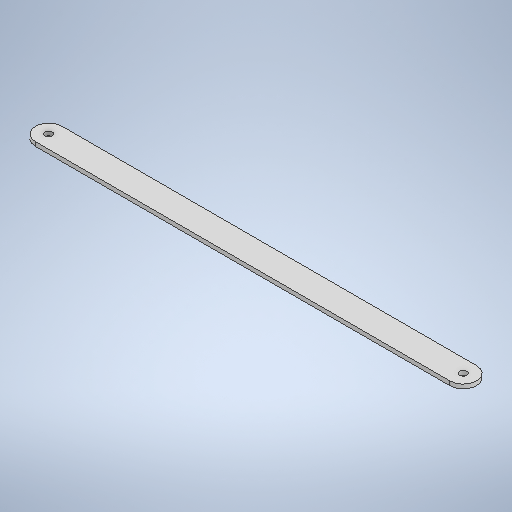
# Autodesk Inventor part: A1P2
Saved by Autodesk Inventor 2025.2 (Build 292293000, 293)
## iProperties
Created: 2025-05-22
Part Number: A1P2
Material: Generic
Document SubType Name: Sheet Metal
Designer: Admin
Density: 1 g/cm^3
Sheet Metal Rule: Default
Appearance: Default
Author: Admin
Autodesk Inventor part; units mm, degrees
ref_plane "YZ Plane" through (0, 0, 0) normal (1, 0, 0) x (0, 1, 0)
ref_plane "XZ Plane" through (0, 0, 0) normal (0, 1, 0) x (-1, 0, 0)
ref_plane "XY Plane" through (0, 0, 0) normal (0, 0, 1) x (1, 0, 0)
sketch "Sketch1" plane through (0, 0, 0) normal (0, 1, 0) x (-1, 0, 0)
  arc A0 (0, 5.4545) -> (0, -5.4545) centre (0, 0) ccw
  arc A1 (170, -5.4545) -> (170, 5.4545) centre (170, 0) ccw
  line L0 (0, 5.4545) -> (170, 5.4545)
  line L1 (170, -5.4545) -> (0, -5.4545)
  dimension "d0" = 10.909
  dimension "d1" = 10.909
  dimension "d2" = 170
  constraints: 4 end point, 4 point on circle, 4 tangent, 2 centre point, 1 coincident
  measures "d0" diameter of A0
  measures "d1" diameter of A1
  measures "d2" distance of point (0, 0) A1.centre
extrude "Extrusion1" add sketch "Sketch1" along normal blind 1.7
sketch "Sketch2" plane through (0, 1.7, 0) normal (0, 1, 0) x (1, 0, 0)
  arc A0 (0, -5.4545) -> (0, 5.4545) centre (0, 0) ccw projected
  arc A1 (-170, 5.4545) -> (-170, -5.4545) centre (-170, 0) ccw projected
  circle A2 centre (0, 0) radius 1.5
  circle A3 centre (-170, 0) radius 1.5
  dimension "d5" = 3
  dimension "d6" = 3
  constraints: 2 centre point, 2 coincident
  measures "d5" diameter of A2
  measures "d6" diameter of A3
extrude "Extrusion2" cut sketch "Sketch2" against normal blind 1.7
equation "\"BendRadius\" = Thickness"
equation "\"BendReliefWidth\" = Thickness"
equation "\"BendReliefDepth\" = 0.5 * Thickness"
equation "\"CornerReliefSize\" = 4 * Thickness"
equation "\"MinimumRemnant\" = 2 * Thickness"
equation "\"TransitionRadius\" = BendRadius"
equation "\"JacobiRadiusSize\" = BendRadius"
equation "\"GapSize\" = Thickness"
equation "\"Thickness\" = 3.048"
body "Solid1"
